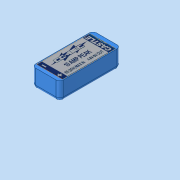
# Autodesk Inventor part: Body
Saved by Autodesk Inventor 2017 (Build 210142000, 142)
## iProperties
Created: 2017-05-21
Part Number: Body
Material: ABS Plastic
Document SubType Name: Modeling
Designer: Derek Wider
Density: 1.06 g/cm^3
Appearance: Cyan
Author: Derek Wider
Autodesk Inventor part; units mm, degrees
ref_plane "YZ Plane" through (0, 0, 0) normal (1, 0, 0) x (0, 1, 0)
ref_plane "XZ Plane" through (0, 0, 0) normal (0, 1, 0) x (-1, 0, 0)
ref_plane "XY Plane" through (0, 0, 0) normal (0, 0, 1) x (1, 0, 0)
sketch "Sketch1" plane through (0, 0, 0) normal (0, 1, 0) x (-1, 0, 0)
  line L0 (0, 0) -> (15, 0)
  line L1 (15, 0) -> (15, -33)
  line L2 (15, -33) -> (0, -33)
  line L3 (0, -33) -> (0, 0)
  dimension "d0" = 15
  dimension "d1" = 33
  constraints: 8 end point, 2 parallel, 1 horizontal, 1 perpendicular
  measures "d0" distance of L1.end L2.end
  measures "d1" distance of L0.end L1.end
extrude "Extrusion1" add sketch "Sketch1" along normal blind 10
fillet "Fillet1" radius 2 2 edges at (0, 0, -16.5) (-15, 0, -16.5)
fillet "Fillet2" radius 2 10 edges at (-0.5858, 0.5858, -33) (-7.5, 0, -33) (-14.4142, 0.5858, -33) (-15, 6, -33) (0, 6, -33) (-0.5858, 0.5858, 0) (-7.5, 0, 0) (-14.4142, 0.5858, 0) (-15, 6, 0) (0, 6, 0)
sketch "Sketch2" plane through (0, 10, 0) normal (0, 1, 0) x (1, 0, 0)
  line L0 (-14.5243, 2) -> (-14.5243, 30.9154) construction
  line L1 (-14.5243, 30.9154) -> (-0.4504, 30.9154) construction
  line L2 (-0.4504, 30.9154) -> (-0.4504, 2) construction
  line L3 (-0.4504, 2) -> (-14.5243, 2) construction
  constraints: 1 vertical, 2 other
body "Solid1"
